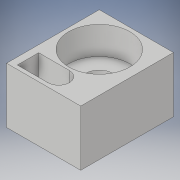
# Autodesk Inventor part: BoitCase
Saved by Autodesk Inventor 2019 (Build 230136000, 136)
## iProperties
Created: 2019-04-08
Part Number: BoitCase
Material: Generic
Document SubType Name: Modeling
Designer: Jorian Brusind
Density: 1 g/cm^3
Appearance: Default
Author: Jorian Brusind
Autodesk Inventor part; units mm, degrees
ref_plane "YZ Plane" through (0, 0, 0) normal (1, 0, 0) x (0, 1, 0)
ref_plane "XZ Plane" through (0, 0, 0) normal (0, 1, 0) x (-1, 0, 0)
ref_plane "XY Plane" through (0, 0, 0) normal (0, 0, 1) x (1, 0, 0)
sketch "Sketch1" plane through (0, 0, 0) normal (0, 1, 0) x (-1, 0, 0)
  line L0 (0, 0) -> (80, 0)
  line L1 (80, 0) -> (80, -100)
  line L2 (80, -100) -> (0, -100)
  line L3 (0, -100) -> (0, 0)
  dimension "d0" = 80
  dimension "d1" = 100
  constraints: 8 end point, 2 parallel, 1 horizontal, 1 perpendicular
  measures "d0" distance of L1.end L2.end
  measures "d1" distance of L0.end L1.end
extrude "Extrusion1" add sketch "Sketch1" along normal blind 60
sketch "Sketch2" plane through (0, 60, 0) normal (0, 1, 0) x (1, 0, 0)
  line L0 (-80, 100) -> (-80, 0) projected
  line L1 (-80, 0) -> (-43, 0)
  line L2 (-80, 0) -> (0, 0) projected
  line L3 (-43, 0) -> (-43, 63)
  circle A0 centre (-43, 63) radius 33
  line L4 (-43, 0) -> (-43, 15)
  dimension "d4" = 37
  dimension "d5" = 63
  dimension "d6" = 66
  constraints: 6 end point, 2 point on line, 1 centre point, 1 coincident, 1 perpendicular
  measures "d4" distance of L0.end L1.end
  measures "d5" distance of L1.end L3.end
  measures "d6" diameter of A0
extrude "Extrusion2" cut sketch "Sketch2" against normal blind 30
sketch "Sketch3" plane through (-43, 30, -63) normal (0, 1, 0) x (1, 0, 0)
  circle A0 centre (0, 0) radius 15
  line L0 (43, 37) -> (-37, 37) projected
  line L1 (-37, 37) -> (-37, -63) projected
  point P0 (43, -63)
  dimension "d11" = 30
  dimension "d12" = 37
  dimension "d13" = 37
  constraints: 1 centre point
  measures "d11" diameter of A0
  measures "d12" distance from line of L0 A0.centre
  measures "d13" distance from line of L1 A0.centre
extrude "Extrusion3" cut sketch "Sketch3" against normal blind 22
sketch "Sketch4" plane through (-43, 8, -63) normal (0, 1, 0) x (1, 0, 0)
  line L0 (-15, 15) -> (15, 15)
  line L1 (15, 15) -> (15, -58)
  line L2 (15, -58) -> (-15, -58)
  line L3 (-15, -58) -> (-15, 15)
  line L4 (43, 37) -> (-37, 37) projected
  line L5 (43, -63) -> (43, 37) projected
  arc A0 (15, 0) -> (-15, 0) centre (0, 0) ccw
  dimension "d19" = 30
  dimension "d20" = 73
  dimension "d21" = 22
  dimension "d22" = 28
  dimension "d23" = 43
  dimension "d24" = 30
  dimension "d25" = 37
  constraints: 8 end point, 2 parallel, 2 point on circle, 2 point on line, 1 centre point, 1 horizontal, 1 perpendicular
  measures "d19" distance of L1.end L2.end
  measures "d20" distance of L0.end L1.end
  measures "d21" distance between parallel lines of L4 L0
  measures "d22" distance between parallel lines of L5 L1
  measures "d23" distance from line of L5 A0.centre
  measures "d24" diameter of A0
  measures "d25" distance from line of L4 A0.centre
extrude "Extrusion4" cut sketch "Sketch4" along normal mid plane 10 contours A0 L1 L2 L3
sketch "Sketch5" plane through (0, 60, 0) normal (0, 1, 0) x (1, 0, 0)
  circle A0 centre (-39.5, 15.6291) radius 11.5
  line L0 (0, 0) -> (0, 100) projected
  circle A1 centre (-43, 63) radius 33 projected
  line L1 (-39.5, 4.1291) -> (-72.5, 4.1291)
  line L2 (-72.5, 4.1291) -> (-72.5, 27.1291)
  line L3 (-72.5, 27.1291) -> (-39.5, 27.1291)
  line L4 (-39.5, 27.1291) -> (-39.5, 4.1291)
  line L5 (-80, 0) -> (0, 0) projected
  dimension "d28" = 23
  dimension "d29" = 39.5
  dimension "d31" = 33
  dimension "d32" = 33
  dimension "d33" = 23
  dimension "d36" = 15.6291
  constraints: 8 end point, 2 parallel, 1 horizontal, 1 perpendicular, 1 vertical alignment, 2 other
  measures "d29" distance from line of L0 point (-39.5, 15.629)
  measures "d31" distance of L2.end L3.end
  measures "d32" distance from line of L2 point (-39.5, 15.629)
  measures "d33" distance of L1.end L2.end
  measures "d36" distance from line of L5 point (-39.5, 15.629)
extrude "Extrusion5" cut sketch "Sketch5" against normal blind 57 contours A0 L4 | L4 A0 | A0 L1 L2 L3
body "Solid1"
